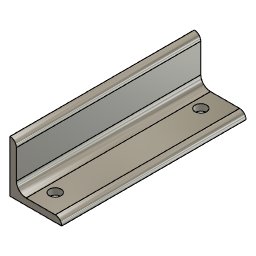
0.880.0051 - Contreplaque - IGTE 21400_18 - Rep. 2 (Autodesk Fusion 360 design; units mm, degrees)
Autodesk Fusion 360 part; units mm, degrees
sketch "Sketch1" plane through (0, 0, 0) normal (0, 0, 1) x (1, 0, 0)
  line L0 (0, 0) -> (80, 0)
  line L1 (0, 0) -> (0, 80)
  line L2 (0, 80) -> (10, 80)
  line L3 (80, 0) -> (80, 10)
  line L4 (10, 80) -> (10, 10)
  line L5 (10, 10) -> (80, 10)
  dimension "d1" = 80
  dimension "d2" = 80
  dimension "d3" = 10
  dimension "d4" = 10
  constraint coincident L0.start L1.start
  constraint perpendicular L0 L4
  measures "d1" distance of L0.start L0.end
  measures "d2" distance of L0.start L1.end
  measures "d3" distance of L1.end L2.end
  measures "d4" distance of L0.end L3.end
extrude "Extrude1" add sketch "Sketch1" along normal mid plane 285
fillet "Fillet1" radius 10 2 edges at (80, 10, 0) (10, 80, 0)
fillet "Fillet2" radius 15 1 edges at (10, 10, 0)
sketch "Sketch2" plane through (0, 0, 0) normal (0, -1, 0) x (1, 0, 0)
  line L0 (80, -142.5) -> (80, 142.5)
  line L1 (80, 142.5) -> (0, 142.5)
  line L2 (0, 142.5) -> (0, -142.5)
  line L3 (0, -142.5) -> (80, -142.5)
  circle A0 centre (40, 112.5) radius 9
  line L4 (25, -142.5) -> (70, -142.5)
  line L5 (40, 142.5) -> (40, -142.5) construction
  line L6 (40, 142.5) -> (40, 112.5) construction
  line L7 (0, 0) -> (80, 0) construction
  circle A1 centre (40, -112.5) radius 9
  dimension "d9" = 18
  dimension "d10" = 30
  constraint midpoint L1 L5.start
  constraint midpoint L3 L5.end
  constraint coincident A0.centre L6.end
  constraint coincident L7.start origin
  constraint midpoint L0 L7.end
  constraint symmetric A0 L7 A1
  measures "d9" diameter of A0
  measures "d10" distance of L5.start A0.centre
extrude "Extrude2" cut sketch "Sketch2" against normal through all contours A0 | A1
